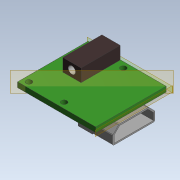
# Autodesk Inventor part: F001-PCB1
Saved by Autodesk Inventor 2020 (Build 240168000, 168)
## iProperties
Created: 2021-07-23
Part Number: F001-PCB1
Material: Générique
Document SubType Name: Modeling
Designer: gregory.trottet
Density: 1 g/cm^3
Appearance: Par défaut
Author: gregory.trottet
Autodesk Inventor part; units mm, degrees
ref_plane "YZ Plane" through (0, 0, 0) normal (1, 0, 0) x (0, 1, 0)
ref_plane "XZ Plane" through (0, 0, 0) normal (0, 1, 0) x (-1, 0, 0)
ref_plane "XY Plane" through (0, 0, 0) normal (0, 0, 1) x (1, 0, 0)
sketch "Sketch1" plane through (0, 0, 0) normal (0, 0, 1) x (1, 0, 0)
  line L0 (0, 0) -> (-27.7, 0)
  line L1 (-27.7, 0) -> (-27.7, 25)
  line L2 (-27.7, 25) -> (0, 25)
  line L3 (0, 25) -> (0, 0)
  circle A0 centre (-25.7, 23) radius 1
  circle A1 centre (-13.2, 23) radius 1
  circle A2 centre (-13.2, 2) radius 1
  circle A3 centre (-25.7, 2) radius 1
  line L4 (-25.7, 2) -> (-25.7, 23) construction
  line L5 (-25.7, 23) -> (-13.2, 23) construction
  line L6 (-13.2, 23) -> (-13.2, 2) construction
  line L7 (-13.2, 2) -> (-25.7, 2) construction
  line L8 (-13.2, 12.5) -> (0, 12.5) construction
  dimension "d0" = 25
  dimension "d1" = 27.7
  dimension "d2" = 12.5
  dimension "d3" = 21
  dimension "d4" = 2
  dimension "d5" = 2
  constraints: 18 end point, 4 centre point, 3 equal radius, 3 parallel, 3 perpendicular, 2 horizontal, 2 midpoint, 1 vertical
  measures "d0" distance of L2.end L0.start
  measures "d1" distance of L1.end L2.end
  measures "d2" distance of L4.end L5.end
  measures "d3" distance of L5.end L6.end
  measures "d4" distance between parallel lines of L1 L4
  measures "d5" diameter of A1
extrude "Extrusion1" add sketch "Sketch1" along normal blind 1.8
sketch "Sketch2" plane through (0, 0, 1.8) normal (0, 0, 1) x (1, 0, 0)
  line L0 (0, 0) -> (0, 25) construction
  line L1 (0, 25) -> (-27.7, 25) construction
  line L2 (-27.7, 25) -> (-27.7, 0) construction
  line L3 (-27.7, 0) -> (0, 0) construction
  circle A0 centre (-25.7, 2) radius 1 construction
  circle A1 centre (-13.2, 2) radius 1 construction
  circle A2 centre (-13.2, 23) radius 1 construction
  circle A3 centre (-25.7, 23) radius 1 construction
  line L4 (-22.7, 11) -> (-16.2, 11)
  line L5 (-16.2, 11) -> (-16.2, 24.9)
  line L6 (-16.2, 24.9) -> (-22.7, 24.9)
  line L7 (-22.7, 24.9) -> (-22.7, 11)
  dimension "d8" = 6.5
  dimension "d10" = 5
  dimension "d33" = 14
  dimension "d34" = 0.1
  constraints: 8 end point, 2 parallel, 1 horizontal, 1 perpendicular
  measures "d8" distance of L5.end L6.end
  measures "d10" distance between parallel lines of L2 L7
  measures "d33" distance between parallel lines of L1 L4
  measures "d34" distance between parallel lines of L1 L6
extrude "Extrusion2" add sketch "Sketch2" along normal blind 4.5
ref_plane "Work Plane1" through (0, 25, 0) normal (0.7071, -0.7071, 0) x (0, 0, -1)
ref_plane "Work Plane2" through (-27.7, 26, 0) normal (0, 1, 0) x (1, 0, 0)
ref_plane "Work Plane3" through (1, 0, 0) normal (1, 0, 0) x (0, 0, -1)
sketch "Sketch4" plane through (1, 0, 0) normal (1, 0, 0) x (0, 0, -1)
  line L0 (5.5, 20) -> (3, 20)
  line L1 (0.5, 17.5) -> (0.5, 7.5)
  line L2 (3, 5) -> (5.5, 5)
  line L3 (6, 5.5) -> (6, 19.5)
  line L4 (0, 0) -> (0, 25) construction
  line L5 (2.6464, 19.8536) -> (0.6464, 17.8536)
  line L6 (2.6464, 5.1464) -> (0.6464, 7.1464)
  line L7 (6, 12.5) -> (0, 12.5) construction
  arc A0 (6, 19.5) -> (5.5, 20) centre (5.5, 19.5) ccw
  arc A1 (5.5, 5) -> (6, 5.5) centre (5.5, 5.5) ccw
  arc A2 (2.6464, 5.1464) -> (3, 5) centre (3, 5.5) ccw
  arc A3 (0.5, 7.5) -> (0.6464, 7.1464) centre (1, 7.5) ccw
  arc A4 (0.6464, 17.8536) -> (0.5, 17.5) centre (1, 17.5) ccw
  arc A5 (3, 20) -> (2.6464, 19.8536) centre (3, 19.5) ccw
  line L8 (5.5, 19.5) -> (5.5, 5.5)
  line L9 (5.5, 5.5) -> (3, 5.5)
  line L10 (3, 5.5) -> (1, 7.5)
  line L11 (1, 7.5) -> (1, 17.5)
  line L12 (1, 17.5) -> (3, 19.5)
  line L13 (3, 19.5) -> (5.5, 19.5)
  point P0 (6, 20)
  point P1 (6, 5)
  point P2 (0.5, 12.5)
  dimension "d17" = 0.5
  dimension "d19" = 15
  dimension "d20" = 5.5
  dimension "d21" = 0.5
  dimension "d22" = 135
  dimension "d23" = 3
  dimension "d24" = 0.5
  constraints: 26 end point, 12 point on circle, 12 tangent, 6 centre point, 5 equal radius, 5 point on line, 4 parallel, 3 midpoint, 3 perpendicular, 2 horizontal, 5 other
  measures "d17" distance between parallel lines of L4 L1
  measures "d19" distance of point (6, 5) point (6, 20)
  measures "d20" distance between parallel lines of L3 L1
  measures "d21" radius of A0
  measures "d22" angle of L0 L5
  measures "d23" distance from line of L2.start L3
  measures "d24" distance between parallel lines of L3 L8
extrude "Extrusion3" add sketch "Sketch4" against normal blind 10.5
sketch "Sketch5" plane through (1, 5.5, -6) normal (0, 0, -1) x (-1, 0, 0)
  line L0 (1, -5.5) -> (1, 19.5) construction
  line L1 (28.7, -5.5) -> (1, -5.5) construction
  line L2 (28.7, 19.5) -> (28.7, -5.5) construction
  line L3 (1, 19.5) -> (28.7, 19.5) construction
  circle A0 centre (26.7, -3.5) radius 1 construction
  circle A1 centre (14.2, -3.5) radius 1 construction
  circle A2 centre (14.2, 17.5) radius 1 construction
  circle A3 centre (26.7, 17.5) radius 1 construction
  line L4 (0, 0) -> (0, 14) construction
  line L5 (0, 0) -> (10.5, 0) construction
  line L6 (10.5, 14) -> (10.5, 0) construction
  line L7 (0, 14) -> (10.5, 14) construction
  line L8 (0, -0.5) -> (10.5, -0.5) construction
  line L9 (1, -5.5) -> (1, 19.5) construction
  line L10 (28.7, -5.5) -> (1, -5.5) construction
  line L11 (28.7, 19.5) -> (28.7, -5.5) construction
  line L12 (1, 19.5) -> (28.7, 19.5) construction
  circle A4 centre (26.7, -3.5) radius 1 construction
  circle A5 centre (14.2, -3.5) radius 1 construction
  circle A6 centre (14.2, 17.5) radius 1 construction
  circle A7 centre (26.7, 17.5) radius 1 construction
  line L13 (0, 14.5) -> (10.5, 14.5) construction
  line L14 (12.2, 14.5) -> (7.1495, 14.5)
  line L15 (7.1495, 14.5) -> (7.1495, 14)
  line L16 (7.1495, 14) -> (12.2, 14)
  line L17 (12.2, 14) -> (12.2, 14.5)
  line L18 (12.2, -0.5) -> (7.1495, -0.5)
  line L19 (7.1495, -0.5) -> (7.1495, 0)
  line L20 (7.1495, 0) -> (12.2, 0)
  line L21 (12.2, 0) -> (12.2, -0.5)
  dimension "d27" = 12.2
  constraints: 18 end point, 6 point on line, 4 centre point, 4 parallel, 2 horizontal, 2 perpendicular
  measures "d27" distance between parallel lines of L17 L4
extrude "Extrusion4" add sketch "Sketch5" against normal up to surface (6 mm away)
sketch "Sketch6" plane through (-22.7, 11, 1.8) normal (0, -1, 0) x (1, 0, 0)
  line L0 (6.5, 0) -> (0, 0) construction
  line L1 (6.5, 0) -> (6.5, 4.5) construction
  line L2 (0, 4.5) -> (6.5, 4.5) construction
  line L3 (0, 0) -> (0, 4.5) construction
  line L4 (6.5, 0) -> (0, 4.5)
  circle A0 centre (3.25, 2.25) radius 1.3
  point P0 (22.7, -1.8)
  dimension "d30" = 2.6
  constraints: 2 end point, 2 midpoint, 1 centre point
  measures "d30" diameter of A0
extrude "Extrusion5" cut sketch "Sketch6" against normal through all
body "Solid1"
